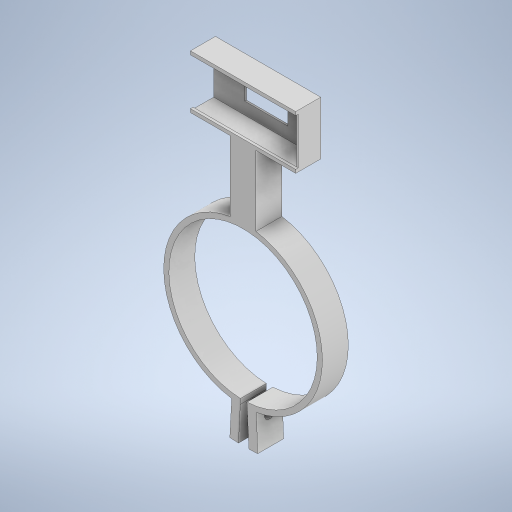
# Autodesk Inventor part: camera_robotarm2
Saved by Autodesk Inventor 2024.3 (Build 283343000, 343)
## iProperties
Created: 2025-09-30
Part Number: camera_robotarm2
Material: 일반
Document SubType Name: Modeling
Designer: joung
Density: 1 g/cm^3
Appearance: 기본값
Author: joung
Autodesk Inventor part; units mm, degrees
ref_plane "YZ Plane" through (0, 0, 0) normal (1, 0, 0) x (0, 1, 0)
ref_plane "XZ Plane" through (0, 0, 0) normal (0, 1, 0) x (-1, 0, 0)
ref_plane "XY Plane" through (0, 0, 0) normal (0, 0, 1) x (1, 0, 0)
sketch "스케치1" plane through (0, 0, 0) normal (0, 0, 1) x (1, 0, 0)
  line L0 (-29.5, 14.5) -> (29.5, 14.5)
  line L1 (29.5, 14.5) -> (29.5, -14.5)
  line L2 (29.5, -14.5) -> (-29.5, -14.5)
  line L3 (-29.5, -14.5) -> (-29.5, 14.5)
  line L4 (-29.5, 14.5) -> (29.5, -14.5) construction
  line L5 (29.5, 14.5) -> (-29.5, -14.5) construction
  line L6 (30.5, 15.5) -> (-30.5, 15.5)
  line L7 (-30.5, 15.5) -> (-30.5, -15.5)
  line L8 (-30.5, -15.5) -> (30.5, -15.5)
  line L9 (30.5, -15.5) -> (30.5, 15.5)
  point P0 (0, 0)
  dimension "d0" = 59
  dimension "d1" = 29
  dimension "d4" = 1
  constraints: 20 end point, 4 parallel, 2 midpoint, 2 perpendicular, 1 horizontal, 3 other
  measures "d0" distance of L1.end L2.end
  measures "d1" distance of L0.end L1.end
  measures "d4" distance between parallel lines of L0 L6
extrude "돌출1" add sketch "스케치1" along normal blind 1 contours L0 L1 L2 L3 | L9 L8 L7 L6
sketch "스케치2" plane through (0, 0, 1) normal (0, 0, 1) x (1, 0, 0)
  line L0 (30.5, -15.5) -> (30.5, 15.5) projected
  line L1 (-30.5, -15.5) -> (30.5, -15.5)
  line L2 (30.5, -15.5) -> (30.5, 15.5)
  line L3 (30.5, 15.5) -> (-30.5, 15.5)
  line L4 (-30.5, 15.5) -> (-30.5, -15.5)
  line L5 (-30.5, -15.5) -> (30.5, 15.5) construction
  line L6 (30.5, -15.5) -> (-30.5, 15.5) construction
  line L7 (-29.5, 14.5) -> (29.5, 14.5)
  line L8 (29.5, 14.5) -> (29.5, -14.5)
  line L9 (29.5, -14.5) -> (-29.5, -14.5)
  line L10 (-29.5, -14.5) -> (-29.5, 14.5)
  point P0 (2.95, 1.45)
  dimension "d5" = 1
  constraints: 20 end point, 4 parallel, 2 perpendicular, 1 horizontal, 3 other
  measures "d5" distance between parallel lines of L3 L7
extrude "돌출2" add sketch "스케치2" along normal blind 12
sketch "스케치3" plane through (0, 0, 1) normal (0, 0, 1) x (1, 0, 0)
  line L0 (-12.5, -7.5) -> (12.5, -7.5)
  line L1 (12.5, -7.5) -> (12.5, 7.5)
  line L2 (12.5, 7.5) -> (-12.5, 7.5)
  line L3 (-12.5, 7.5) -> (-12.5, -7.5)
  line L4 (-12.5, -7.5) -> (12.5, 7.5) construction
  line L5 (12.5, -7.5) -> (-12.5, 7.5) construction
  point P0 (0, 0)
  dimension "d8" = 25
  dimension "d9" = 15
  constraints: 12 end point, 2 midpoint, 2 parallel, 1 horizontal, 1 perpendicular
  measures "d8" distance of L2.end L1.end
  measures "d9" distance of L1.end L0.end
extrude "돌출3" cut sketch "스케치3" against normal blind 12
sketch "스케치4" plane through (-30.5, -15.5, 0) normal (-1, 0, 0) x (0, 0, 1)
  line L0 (1, 30) -> (13, 30) projected
  line L1 (1, 1) -> (1, 30) projected
  line L2 (13, 30) -> (1, 30)
  line L3 (1, 30) -> (1, 1)
  line L4 (1, 1) -> (13, 1)
  line L5 (13, 1) -> (13, 30)
  point P0 (0, 15.5)
  constraints: 8 end point, 2 parallel, 1 horizontal, 1 perpendicular
extrude "돌출4" cut sketch "스케치4" against normal blind 15
sketch "스케치5" plane through (-30.5, -15.5, 0) normal (-1, 0, 0) x (0, 0, 1)
  line L0 (13, 0) -> (13, 31) projected
  line L1 (13, 31) -> (14.5, 31)
  line L2 (14.5, 31) -> (14.5, 29)
  line L3 (14.5, 29) -> (13, 29)
  line L4 (13, 29) -> (13, 31)
  line L5 (13, 0) -> (14.5, 0)
  line L6 (14.5, 0) -> (14.5, 2)
  line L7 (14.5, 2) -> (13, 2)
  line L8 (13, 2) -> (13, 0)
  point P0 (0, 15.5)
  point P1 (13, 2)
  dimension "d14" = 1.5
  dimension "d15" = 2
  dimension "d16" = 2
  constraints: 16 end point, 4 parallel, 2 horizontal, 2 perpendicular, 1 point on line
  measures "d14" distance of L2.end L3.end
  measures "d15" distance of L1.end L2.end
  measures "d16" distance of L6.end L5.end
extrude "돌출5" add sketch "스케치5" against normal up to surface (61 mm away)
sketch "스케치6" plane through (-30.5, -15.5, 0) normal (0, -1, 0) x (1, 0, 0)
  line L0 (0, 14.5) -> (61, 14.5) projected
  line L1 (23, -0.5) -> (38, -0.5)
  line L2 (38, -0.5) -> (38, 14.5)
  line L3 (38, 14.5) -> (23, 14.5)
  line L4 (23, 14.5) -> (23, -0.5)
  line L5 (23, -0.5) -> (38, 14.5) construction
  line L6 (38, -0.5) -> (23, 14.5) construction
  point P0 (30.5, 0)
  point P1 (30.5, 7)
  dimension "d19" = 15
  constraints: 12 end point, 2 midpoint, 2 parallel, 1 horizontal, 1 perpendicular, 1 point on line
  measures "d19" distance of L3.end L2.end
extrude "돌출6" add sketch "스케치6" along normal blind 40
sketch "스케치7" plane through (-30.5, -13.5, 14.5) normal (0, 0, 1) x (1, 0, 0)
  line L0 (38, -42) -> (23, -42) projected
  line L1 (30.5, -42) -> (30.5, -88)
  circle A0 centre (30.5, -88) radius 46
  circle A1 centre (30.5, -88) radius 43
  line L2 (23, -42) -> (23, -42.6155)
  line L3 (38, -2) -> (38, -42) projected
  line L4 (38, -42) -> (38, -42.6155)
  line L5 (30.5, -88) -> (32.9075, -133.937)
  line L6 (30.5, -88) -> (76.5, -88) construction
  line L7 (30.5, -88) -> (28.8946, -133.972)
  line L8 (28.8946, -133.972) -> (27.8479, -153.9446)
  line L9 (28.8946, -133.972) -> (48.8946, -133.972) construction
  line L10 (32.9075, -133.937) -> (33.9542, -153.9095)
  line L11 (32.9075, -133.937) -> (52.9075, -133.937) construction
  line L12 (33.9542, -153.9095) -> (38.9511, -153.7351)
  line L13 (33.9542, -153.9095) -> (38.9542, -153.9095) construction
  line L14 (38.9511, -153.7351) -> (38.2598, -133.937)
  line L15 (27.8479, -153.9446) -> (29.0856, -153.9446) construction
  line L16 (38.2598, -133.937) -> (38.2391, -133.3443)
  line L17 (27.8479, -153.9446) -> (22.8548, -153.6829)
  line L18 (27.8479, -153.9446) -> (32.8479, -153.9446) construction
  line L19 (22.8548, -153.6829) -> (23.9112, -133.5257)
  point P0 (30.5, 13.5)
  point P1 (27.1993, -133.8814)
  point P2 (32.7504, -130.9411)
  point P3 (28.9993, -130.9738)
  dimension "d22" = 46
  dimension "d23" = 3
  dimension "d24" = 87
  dimension "d25" = 20
  dimension "d26" = 93
  dimension "d27" = 20
  dimension "d28" = 87
  dimension "d29" = 5
  dimension "d30" = 2
  dimension "d31" = 90
  dimension "d42" = 5
  dimension "d43" = 177
  dimension "d44" = 90
  constraints: 36 end point, 6 horizontal, 5 equal length, 2 collinear, 2 point on line, 2 vertical, 1 centre point, 1 coincident, 1 midpoint, 10 other
  measures "d22" distance of L1.start L1.end
  measures "d24" angle of L5 L6
  measures "d25" distance of L7.end L8.end
  measures "d26" angle of L8 L9
  measures "d27" distance of L5.end L10.end
  measures "d28" angle of L10 L11
  measures "d29" distance of L10.end L12.end
  measures "d30" angle of L13 L12
  measures "d31" angle of L14 L12
  measures "d42" distance of L8.end L17.end
  measures "d43" angle of L18 L17
  measures "d44" angle of L17 L19
extrude "돌출7" add sketch "스케치7" against normal up to surface (15 mm away) contours L4 A0 L0 | A0 L2 L0 | A0 L5 A1 L1 | L1 A1 L7 A0 | A0 L8 L17 L19 | L16 L14 L12 L10 A0
sketch "스케치9" plane through (7.7391, -146.8443, 14.5) normal (0.9994, 0.0349, 0) x (0, 0, -1)
  line L0 (0, -20.2251) -> (0, 2.6915) projected
  line L1 (0, -8.7668) -> (15, 1.1952)
  line L2 (15, -0.3012) -> (15, 2.6915) projected
  circle A0 centre (7.5, -3.7858) radius 3.1
  point P0 (14.5, 147.025)
  point P1 (15, -19.971)
  dimension "d39" = 6.2
  constraints: 3 midpoint, 2 end point, 1 centre point
  measures "d39" diameter of A0
extrude "돌출9" cut sketch "스케치9" against normal blind 10
sketch "스케치10" plane through (-7.6452, -167.1829, -0.5) normal (-0.9986, 0.0523, 0) x (0, 0, 1)
  line L0 (15, 0) -> (0, 0) projected
  line L1 (7.5, 0) -> (7.5, 11.7)
  circle A0 centre (7.5, 11.7) radius 3.1
  point P0 (0.5, 167.3539)
  dimension "d45" = 11.7
  dimension "d46" = 6.2
  constraints: 2 end point, 1 centre point, 1 coincident, 1 midpoint, 1 vertical
  measures "d45" distance of L1.start L1.end
  measures "d46" diameter of A0
extrude "돌출10" cut sketch "스케치10" against normal up to surface (5 mm away)
